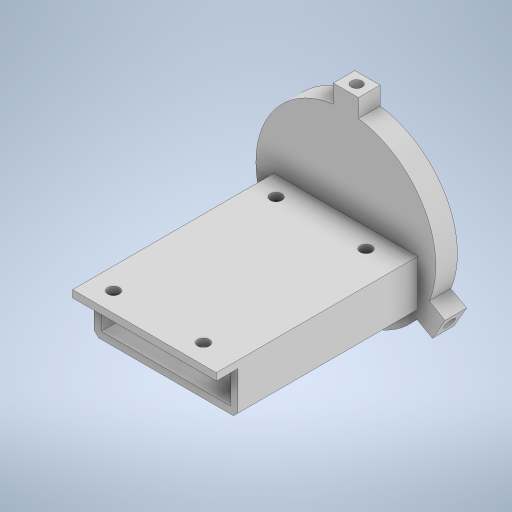
# Autodesk Inventor part: Electronic casing
Saved by Autodesk Inventor 2024 (Build 280153000, 153)
## iProperties
Created: 2024-03-27
Part Number: Electronic casing
Material: Generic
Document SubType Name: Modeling
Designer: auror
Density: 1 g/cm^3
Appearance: Default
Author: auror
Autodesk Inventor part; units mm, degrees
ref_plane "YZ Plane" through (0, 0, 0) normal (1, 0, 0) x (0, 1, 0)
ref_plane "XZ Plane" through (0, 0, 0) normal (0, 1, 0) x (-1, 0, 0)
ref_plane "XY Plane" through (0, 0, 0) normal (0, 0, 1) x (1, 0, 0)
sketch "Sketch2" plane through (0, 0, 0) normal (0, 1, 0) x (-1, 0, 0)
  line L0 (18.5, 28) -> (-21.5, 28)
  line L1 (-21.5, 28) -> (-21.5, -28)
  line L2 (-21.5, -28) -> (18.5, -28)
  line L3 (18.5, -28) -> (18.5, 28)
  point P0 (0, 0)
  point P1 (-21.5, 0)
  point P2 (18.5, 0)
  dimension "d0" = 40
  dimension "d1" = 56
  dimension "d2" = 28
  dimension "d3" = 18.5
  constraints: 8 end point, 2 midpoint, 2 parallel, 1 horizontal, 1 perpendicular
  measures "d0" distance of point (-21.5, 0) point (18.5, 0)
  measures "d1" distance between parallel lines of L2 L0
  measures "d2" distance from line of point (0, 0) L0
  measures "d3" distance from line of L3 point (0, 0)
extrude "Extrusion1" add sketch "Sketch2" along normal blind 2
sketch "Sketch3" plane through (0, 2, 0) normal (0, 1, 0) x (1, 0, 0)
  circle A0 centre (12.5, -22.6) radius 1.6
  circle A1 centre (-12.5, -22.6) radius 1.6
  circle A2 centre (-12.5, 22.6) radius 1.6
  circle A3 centre (12.5, 22.6) radius 1.6
  point P0 (0, 0)
  dimension "d7" = 12.5
  dimension "d8" = 3.2
  dimension "d9" = 3.2
  dimension "d10" = 3.2
  dimension "d11" = 3.2
  dimension "d65" = 25
  dimension "d66" = 25
  dimension "d67" = 45.2
  dimension "d68" = 0
  dimension "d69" = 45.2
  dimension "d70" = 0
  dimension "d71" = 12.5
  dimension "d72" = 22.6
  constraints: 4 centre point, 4 coincident
  measures "d7" horizontal distance of point (0, 0) point (12.5, -22.6)
  measures "d8" diameter of A0
  measures "d9" diameter of A1
  measures "d10" diameter of A2
  measures "d11" diameter of A3
  measures "d65" distance of A3.centre point (-12.5, 22.6)
  measures "d66" distance of A0.centre A1.centre
  measures "d67" distance of A1.centre A2.centre
  measures "d68" horizontal distance of A1.centre A2.centre
  measures "d69" distance of A0.centre A3.centre
  measures "d70" vertical distance of A3.centre A2.centre
  measures "d71" horizontal distance of point (0, 0) A2.centre
  measures "d72" vertical distance of point (0, 0) A3.centre
hole "Hole1" at (12.5, 2, 22.6) at (-12.5, 2, 22.6) at (-12.5, 2, -22.6) at (12.5, 2, -22.6) direction (0, -1, 0) diameter 3.2 end through all
sketch "Sketch4" plane through (21.5, 0, -28) normal (0, 0, -1) x (-1, 0, 0)
  line L0 (20, 27.2049) -> (20, 0.4053) construction
  line L1 (20, 2.2049) -> (7.2369, -5.1639) construction
  line L2 (20, 2.2049) -> (20, 27.2049) construction
  line L3 (20, 2.2049) -> (41.6506, -10.2951) construction
  line L4 (16.5, 32) -> (16.5, 26.9587)
  line L5 (23.5, 32) -> (23.5, 26.9587)
  line L6 (16.5, 32) -> (23.5, 32)
  line L7 (-7.5685, -9.6413) -> (-3.1779, -7.1645)
  line L8 (-4.0623, -15.6999) -> (0.3283, -13.2231)
  line L9 (-7.5685, -9.6413) -> (-4.0623, -15.6999)
  line L10 (43.1867, -7.1428) -> (47.5542, -9.6599)
  line L11 (39.6862, -13.2047) -> (44.0538, -15.7218)
  line L12 (44.0538, -15.7218) -> (47.5542, -9.6599)
  line L13 (20, 2.2049) -> (7.2369, -5.1639) construction
  line L14 (37.68, 12.4124) -> (7.2369, -5.1639) construction
  line L15 (20, 2.2049) -> (20, 27.2049) construction
  line L16 (20, 48.4448) -> (20, 27.2049) construction
  line L17 (20, 2.2049) -> (41.6506, -10.2951) construction
  line L18 (78.0931, -31.3352) -> (41.6506, -10.2951) construction
  arc A0 (0.3283, -13.2231) -> (39.6862, -13.2047) centre (20, 2.2049) ccw
  arc A1 (16.5, 26.9587) -> (-3.1779, -7.1645) centre (20, 2.2049) ccw
  arc A2 (43.1867, -7.1428) -> (23.5, 26.9587) centre (20, 2.2049) ccw
  line L19 (44.9992, 2) -> (-4.9992, 2) construction
  line L20 (40, 2) -> (0, 2) projected
  point P0 (21.5, 0)
  point P1 (-1.867, -14.4615)
  point P2 (41.87, -14.4632)
  point P3 (-5.3732, -8.4029)
  point P4 (23.5, 29.4793)
  point P5 (45.3705, -8.4013)
  point P6 (20, 32)
  dimension "d32" = 7
  dimension "d33" = 7
  dimension "d34" = 7
  dimension "d37" = 3.5
  dimension "d38" = 3.5
  dimension "d39" = 3.5
  dimension "d40" = 5.0414
  dimension "d45" = 120
  dimension "d46" = 120
  dimension "d49" = 5.0414
  dimension "d51" = 5.041
  dimension "d52" = 5.041
  dimension "d53" = 5.041
  dimension "d54" = 5.041
  dimension "d55" = 7
  dimension "d56" = 7
  dimension "d57" = 7
  dimension "d58" = 25
  dimension "d59" = 25
  dimension "d60" = 25
  dimension "d63" = 30
  dimension "d64" = 0
  dimension "d84" = 20
  constraints: 40 end point, 17 point on circle, 6 midpoint, 5 collinear, 3 centre point, 3 point on line, 1 coincident, 1 horizontal, 1 vertical
  measures "d32" distance of point (-1.867, -14.462) point (-5.373, -8.403)
  measures "d33" distance from line of point (23.5, 29.479) L4
  measures "d34" distance of point (45.37, -8.401) point (41.87, -14.463)
  measures "d37" distance from line of L14 point (-1.867, -14.462)
  measures "d38" distance from line of point (23.5, 29.479) L16
  measures "d39" distance from line of L18 point (45.37, -8.401)
  measures "d40" distance of L4.start L4.end
  measures "d45" angle of L17 L2
  measures "d46" angle of L3 L14
  measures "d49" distance of L5.start L5.end
  measures "d51" distance of L7.start L7.end
  measures "d52" distance of L8.start L8.end
  measures "d53" distance of L10.end L10.start
  measures "d54" distance of L11.start L11.end
  measures "d55" distance of L8.end L7.end
  measures "d56" distance of L10.start L11.start
  measures "d57" distance of L5.end L4.end
  measures "d58" radius of A2
  measures "d59" radius of A0
  measures "d60" radius of A1
  measures "d63" distance from line of point (20, 32) L19
  measures "d64" distance between parallel lines of L20 L19
  measures "d84" horizontal distance of A0.centre L20.start
extrude "Extrusion2" add sketch "Sketch4" along normal blind 6
sketch "Sketch5" plane through (21.5, 0, -28) normal (0, 0, 1) x (1, 0, 0)
  circle A0 centre (-20, 2.2049) radius 25 construction
  arc A1 (3.1779, -7.1645) -> (-16.5, 26.9587) centre (-20, 2.2049) ccw projected
  line L0 (-16.5, 32) -> (-16.5, 26.9587) projected
  line L1 (-23.5, 32) -> (-16.5, 32) projected
  line L2 (-23.5, 26.9587) -> (-23.5, 32) projected
  arc A2 (-23.5, 26.9587) -> (-43.1867, -7.1428) centre (-20, 2.2049) ccw projected
  line L3 (-47.5542, -9.6599) -> (-43.1867, -7.1428) projected
  line L4 (-44.0538, -15.7218) -> (-47.5542, -9.6599) projected
  line L5 (-39.6862, -13.2047) -> (-44.0538, -15.7218) projected
  arc A3 (-39.6862, -13.2047) -> (-0.3283, -13.2231) centre (-20, 2.2049) ccw projected
  line L6 (4.0623, -15.6999) -> (-0.3283, -13.2231) projected
  line L7 (7.5685, -9.6413) -> (4.0623, -15.6999) projected
  line L8 (3.1779, -7.1645) -> (7.5685, -9.6413) projected
  arc A4 (3.1779, -7.1645) -> (-16.5, 26.9587) centre (-20, 2.2049) ccw projected
  line L9 (0, 0) -> (0, 2) projected
  line L10 (0, 0) -> (-40, 0) projected
  line L11 (-40, 0) -> (-40, 2) projected
  line L12 (0, 2) -> (-40, 2) projected
  line L13 (-2, 0) -> (-38, 0)
  line L14 (-38, 0) -> (-38, -10)
  line L15 (-38, -10) -> (-2, -10)
  line L16 (-2, -10) -> (-2, 0)
  line L17 (-40, -12) -> (0, -12)
  line L18 (0, -12) -> (0, 0)
  line L19 (0, 0) -> (-40, 0)
  line L20 (-40, 0) -> (-40, -12)
  point P0 (-21.5, 0)
  point P1 (-2, 0)
  dimension "d73" = 50
  dimension "d75" = 18
  dimension "d77" = 18
  dimension "d78" = 10
  dimension "d79" = 0
  dimension "d80" = 2
  dimension "d81" = 2
  dimension "d82" = 0
  dimension "d83" = 2
  constraints: 16 end point, 4 parallel, 2 horizontal, 2 perpendicular, 1 centre point, 1 concentric
  measures "d73" diameter of A0
  measures "d75" horizontal distance of A0.centre L13.start
  measures "d77" horizontal distance of A0.centre L14.end
  measures "d78" distance from line of L10 L14.end
  measures "d79" distance from line of L10 L13.start
  measures "d80" horizontal distance of L14.end L17.start
  measures "d81" horizontal distance of L14.end L17.start
  measures "d82" vertical distance of L13.start L18.end
  measures "d83" distance of L13.start L18.end
extrude "Extrusion3" add sketch "Sketch5" along normal blind 50 contours L18 L17 L20 L10 L14 L15 L16
chamfer "Chamfer1" distance 1.25 angle 45 1 edges at (-18.5, -12, -3)
chamfer "Chamfer2" distance 1.25 angle 45 1 edges at (21.5, -12, -3)
sketch "Sketch6" plane through (-2, 32, -28) normal (0, 1, 0) x (1, 0, 0)
  line L0 (0, 0) -> (7, 0) projected
  line L1 (7, 0) -> (7, 6) projected
  point P0 (2, -28)
  point P1 (3.5, 3)
  point P2 (3.5, 0)
  point P3 (7, 3)
  dimension "d93" = 3
  dimension "d94" = 3.5
  constraints: 2 midpoint
  measures "d93" distance of point (3.5, 0) point (3.5, 3)
  measures "d94" distance of point (3.5, 3) point (7, 3)
hole "Hole2" at (1.5, 32, -31) direction (0, -1, 0) diameter 3 depth 10 tip angle 118 counterbore diameter 4 counterbore depth 0
sketch "Sketch7" plane through (25.5623, -15.6999, -28) normal (0.8655164, -0.5008806, 0) x (0, 0, -1)
  line L0 (0, 0) -> (6, 0) projected
  line L1 (0, 7) -> (0, 0) projected
  point P0 (-28, 0.7848)
  point P1 (3, 3.5)
  point P2 (0, 3.5)
  dimension "d102" = 3.5
  dimension "d103" = 3
  constraints: 1 midpoint
  measures "d102" distance from line of L0 point (3, 3.5)
  measures "d103" distance of point (0, 3.5) point (3, 3.5)
hole "Hole3" at (27.3154, -12.6706, -31) direction (-0.8655164, 0.5008806, 0) diameter 3 depth 10 tip angle 118 counterbore diameter 4 counterbore depth 0
sketch "Sketch8" plane through (-26.0542, -9.6599, -34) normal (-0.8659863, -0.5000677, 0) x (0, 0, 1)
  line L0 (6, -7) -> (6, 0) projected
  line L1 (6, -7) -> (0, -7) projected
  point P0 (34, -4.6635)
  point P1 (3, -3.5)
  dimension "d111" = 3
  dimension "d112" = 3.5
  measures "d111" distance from line of L0 point (3, -3.5)
  measures "d112" distance from line of L1 point (3, -3.5)
hole "Hole4" at (-24.304, -12.6909, -31) direction (0.8659863, 0.5000677, 0) diameter 3 depth 10 tip angle 118 counterbore diameter 4 counterbore depth 0
body "Solid1"
